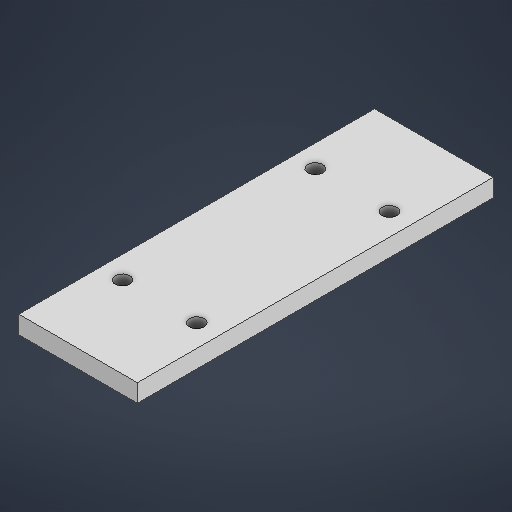
# Autodesk Inventor part: steeringmountplate
Saved by Autodesk Inventor 2026.2 (Build 302298010, 298A)
## iProperties
Created: 2026-07-06
Part Number: steeringmountplate
Material: Generic
Document SubType Name: Modeling
Designer: tasle
Density: 1 g/cm^3
Appearance: Default
Author: tasle
Autodesk Inventor part; units mm, degrees
ref_plane "YZ Plane" through (0, 0, 0) normal (1, 0, 0) x (0, 1, 0)
ref_plane "XZ Plane" through (0, 0, 0) normal (0, 1, 0) x (-1, 0, 0)
ref_plane "XY Plane" through (0, 0, 0) normal (0, 0, 1) x (1, 0, 0)
sketch "Sketch1" plane through (0, 0, 0) normal (0, 1, 0) x (-1, 0, 0)
  line L0 (-17.3414, 16.8049) -> (-57.3414, 16.8049)
  line L1 (-57.3414, 16.8049) -> (-57.3414, -103.1951)
  line L2 (-57.3414, -103.1951) -> (-17.3414, -103.1951)
  line L3 (-17.3414, -103.1951) -> (-17.3414, 16.8049)
  line L4 (-24.8414, -10.6951) -> (-49.8414, -10.6951)
  line L5 (-49.8414, -10.6951) -> (-49.8414, -75.6951)
  line L6 (-49.8414, -75.6951) -> (-24.8414, -75.6951)
  line L7 (-24.8414, -75.6951) -> (-24.8414, -10.6951)
  circle A0 centre (-24.8414, -10.6951) radius 2.5
  circle A1 centre (-24.8414, -75.6951) radius 2.5
  circle A2 centre (-49.8414, -75.6951) radius 2.5
  circle A3 centre (-49.8414, -10.6951) radius 2.5
  point P0 (0, 0)
  dimension "d0" = 40
  dimension "d1" = 120
  dimension "d4" = 25
  dimension "d5" = 65
  dimension "d6" = 27.5
  dimension "d7" = 7.5
  dimension "d8" = 5
  dimension "d9" = 5
  dimension "d10" = 5
  dimension "d11" = 5
  constraints: 16 end point, 4 centre point, 4 coincident, 4 parallel, 2 horizontal, 2 perpendicular
  measures "d0" distance of L2.end L1.end
  measures "d1" distance of L1.end L0.end
  measures "d4" distance of L6.end L5.end
  measures "d5" distance of L5.end L4.end
  measures "d6" distance between parallel lines of L2 L6
  measures "d7" distance between parallel lines of L3 L7
  measures "d8" diameter of A0
  measures "d9" diameter of A1
  measures "d10" diameter of A2
  measures "d11" diameter of A3
extrude "Extrusion1" add sketch "Sketch1" along normal blind 6 contours L3 L2 L1 L0 | L4 A0 L7 A1 L6 A2 L5 A3
body "Solid1"
